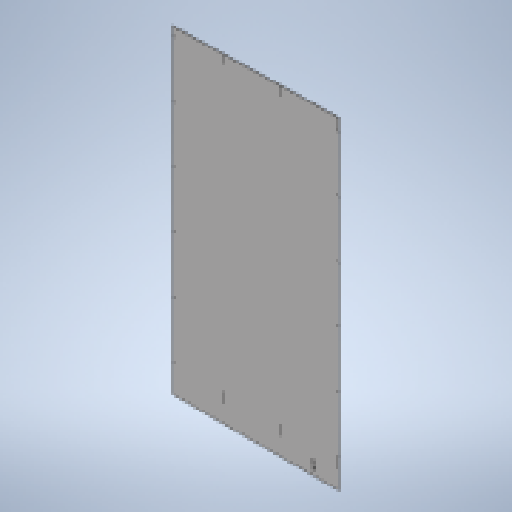
# Autodesk Inventor part: GBK 2231 shield 6
Saved by Autodesk Inventor 2026 (Build 300175000, 175)
## iProperties
Created: 2026-04-17
Part Number: GBK 2231 shield 6
Material: Steel
Document SubType Name: Sheet Metal
Designer: pokla
Stock Number: 2236
Mass: 138487 g
Surface Area: 88564.8 cm^2
Volume: 17641.6 cm^3
Density: 7.85 g/cm^3
Flat Pattern Width: 148 cm
Flat Pattern Length: 284.1 cm
Flat Pattern Area: 42046.8 cm^2
Sheet Metal Rule: По умолчанию_мм
Sheet Metal Width: 1480,000 мм
Sheet Metal Length: 2841,000 мм
Sheet Metal Area: 4204680,000 мм^2
Appearance: Default
Author: admin
Autodesk Inventor part; units mm, degrees
ref_plane "YZ Plane" through (0, 0, 0) normal (1, 0, 0) x (0, 1, 0)
ref_plane "XZ Plane" through (0, 0, 0) normal (0, 1, 0) x (-1, 0, 0)
ref_plane "XY Plane" through (0, 0, 0) normal (0, 0, 1) x (1, 0, 0)
sketch "Sketch1" plane through (0, 0, 0) normal (0, 0, 1) x (1, 0, 0)
  line L0 (740, -1490) -> (-740, -1490)
  line L1 (-740, -1490) -> (-740, 1490)
  line L2 (-740, 1490) -> (740, 1490)
  line L3 (740, 1490) -> (740, -1490)
  line L4 (740, -1490) -> (-740, 1490) construction
  line L5 (-740, -1490) -> (740, 1490) construction
  line L6 (740, 1351) -> (-740, 1317.4141)
  point P0 (0, 0)
  dimension "d0" = 1480
  dimension "d1" = 2980
  dimension "d3" = 1.3
  dimension "d4" = 139
  measures "d0" distance of L1.end L2.end
  measures "d1" distance of L0.end L1.end
  measures "d3" angle of L2 L6
  measures "d4" distance from line of L6.start L2
extrude "Plate1" add sketch "Sketch1" along normal blind 4 contours L0 L1 L6 L3
sketch "Sketch2" plane through (0, 0, 4) normal (0, 0, 1) x (1, 0, 0)
  line L0 (525.5619, -1362.1492) -> (525.5619, -1719.8396) construction
  line L1 (525.5619, -1719.8396) -> (494.2978, -1719.8396) construction
  line L2 (494.2978, -1719.8396) -> (494.2978, -1362.1492) construction
  line L3 (494.2978, -1362.1492) -> (525.5619, -1362.1492) construction
  line L4 (710.2537, -1243.5) -> (710.2537, -1340.5) projected
  line L5 (710.2537, -1340.5) -> (706.2547, -1340.5) projected
  line L6 (210.1251, -1243.5) -> (210.1251, -1340.5) projected
  line L7 (210.1251, -1340.5) -> (206.1261, -1340.5) projected
  line L8 (-290.0035, -1243.5) -> (-290.0035, -1340.5) projected
  line L9 (-290.0035, -1340.5) -> (-294.0025, -1340.5) projected
  line L10 (710.2537, 1454.5) -> (710.2537, 1250.8333) projected
  line L11 (210.1251, 1454.5) -> (210.1251, 1250.8333) projected
  line L12 (-290.0035, 1454.5) -> (-290.0035, 1250.8333) projected
  line L13 (-710, 1247.3333) -> (-739.3197, 1247.3333) projected
  line L14 (-710, 1243.3333) -> (-710, 1247.3333) projected
  line L15 (-710, 750.6667) -> (-739.3197, 750.6667) projected
  line L16 (-710, 746.6667) -> (-710, 750.6667) projected
  line L17 (-710, 254) -> (-739.3197, 254) projected
  line L18 (-710, 250) -> (-710, 254) projected
  line L19 (-710, -242.6667) -> (-739.3197, -242.6667) projected
  line L20 (-710, -246.6667) -> (-710, -242.6667) projected
  line L21 (-710, -739.3333) -> (-739.3197, -739.3333) projected
  line L22 (-710, -743.3333) -> (-710, -739.3333) projected
  line L23 (-710, -1236) -> (-739.3197, -1236) projected
  line L24 (-710, -1240) -> (-710, -1236) projected
  line L25 (770, 1247.3333) -> (710, 1247.3333) projected
  line L26 (710, 1243.3333) -> (710, 1247.3333) projected
  line L27 (770, 750.6667) -> (710, 750.6667) projected
  line L28 (710, 746.6667) -> (710, 750.6667) projected
  line L29 (770, 254) -> (710, 254) projected
  line L30 (710, 250) -> (710, 254) projected
  line L31 (770, -242.6667) -> (710, -242.6667) projected
  line L32 (710, -246.6667) -> (710, -242.6667) projected
  line L33 (770, -739.3333) -> (710, -739.3333) projected
  line L34 (710, -743.3333) -> (710, -739.3333) projected
  line L35 (770, -1236) -> (710, -1236) projected
  line L36 (710, -1240) -> (710, -1236) projected
  point P0 (0, 0)
  constraints: 2 other
mark "Маркировка1"
equation "\"d0\" = Лист_ширина"
equation "\"d2\" = Thickness"
equation "\"BendRadius\" = Thickness"
equation "\"BendReliefWidth\" = Thickness"
equation "\"BendReliefDepth\" = 0.5 * Thickness"
equation "\"CornerReliefSize\" = 4 * Thickness"
equation "\"MinimumRemnant\" = 2 * Thickness"
equation "\"TransitionRadius\" = BendRadius"
equation "\"JacobiRadiusSize\" = BendRadius"
equation "\"GapSize\" = Thickness"
equation "\"Лист_ширина\" = 1480"
equation "\"Thickness\" = 4"
body "Solid1"
